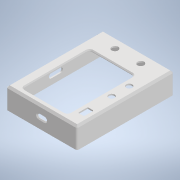
# Autodesk Inventor part: Frontpanel
Saved by Autodesk Inventor 2022 (Build 260153000, 153)
## iProperties
Created: 2020-11-05
Part Number: Frontpanel
Material: Generic
Document SubType Name: Modeling
Designer: simen
Density: 1 g/cm^3
Appearance: Default
Mass: 47.3769 g
Surface Area: 341.342 cm^2
Volume: 47.3769 cm^3
Author: simen
## iProperties of the stored document Frontpanel_3DPrint.ipt
Created: 2022-05-11
Part Number: Frontpanel_3DPrint
Material: Generic
Document SubType Name: Modeling
Designer: simen
Density: 1 g/cm^3
Appearance: Default
Author: simen
Autodesk Inventor part; units mm, degrees
ref_plane "YZ Plane" through (0, 0, 0) normal (1, 0, 0) x (0, 1, 0)
ref_plane "XZ Plane" through (0, 0, 0) normal (0, 1, 0) x (-1, 0, 0)
ref_plane "XY Plane" through (0, 0, 0) normal (0, 0, 1) x (1, 0, 0)
sketch "Sketch1" plane through (0, 0, 0) normal (0, 1, 0) x (-1, 0, 0)
  line L0 (-21.2777, 25.6513) -> (-98.2777, 25.6513)
  line L1 (-98.2777, 25.6513) -> (-98.2777, -79.3487)
  line L2 (-98.2777, -79.3487) -> (-21.2777, -79.3487)
  line L3 (-21.2777, -79.3487) -> (-21.2777, 25.6513)
  point P0 (0, 0)
  dimension "d0" = 77
  dimension "d42" = 105
  constraints: 8 end point, 2 parallel, 1 horizontal, 1 perpendicular
  measures "d0" distance of L2.end L1.end
  measures "d42" distance of L0.end L1.end
extrude "Extrusion1" add sketch "Sketch1" along normal blind 1.5
sketch "Sketch5" plane through (0, 0, 0) normal (0, -1, 0) x (1, 0, 0)
  line L0 (98.2777, 25.6513) -> (98.2777, -79.3487) projected
  line L1 (21.2777, 25.6513) -> (98.2777, 25.6513) projected
  line L2 (21.2777, -79.3487) -> (21.2777, 25.6513) projected
  line L3 (98.2777, -79.3487) -> (21.2777, -79.3487) projected
  line L4 (96.7777, 24.1513) -> (96.7777, -77.8487)
  line L5 (96.7777, -77.8487) -> (22.7777, -77.8487)
  line L6 (22.7777, -77.8487) -> (22.7777, 24.1513)
  line L7 (22.7777, 24.1513) -> (96.7777, 24.1513)
  point P0 (0, 0)
  dimension "d26" = 1.5
  constraints: 8 end point, 3 other
  measures "d26" distance between parallel lines of L1 L7
extrude "Extrusion7" add sketch "Sketch5" along normal blind 21.26
fillet "Fillet2" radius 2 4 edges at (21.2777, -9.88, -79.3487) (98.2777, -9.88, -79.3487) (98.2777, -9.88, 25.6513) (21.2777, -9.88, 25.6513)
sketch "Sketch8" plane through (21.2777, -21.26, -77.3487) normal (-1, 0, 0) x (0, 0, 1)
  line L0 (55.5, 8.76) -> (45.5, 8.76) construction
  line L1 (55.5, 11.26) -> (45.5, 11.26)
  line L2 (45.5, 6.26) -> (55.5, 6.26)
  arc A0 (55.5, 6.26) -> (55.5, 11.26) centre (55.5, 8.76) ccw
  arc A1 (45.5, 11.26) -> (45.5, 6.26) centre (45.5, 8.76) ccw
  line L3 (101, 0) -> (0, 0) projected
  line L4 (101, 0) -> (0, 0) construction
  line L5 (46.5661, 0) -> (44.4339, 17.52) construction
  line L6 (0, 22.76) -> (101, 22.76) projected
  line L7 (0, 22.76) -> (101, 22.76) construction
  line L8 (0, 0) -> (0, 22.76) construction
  line L9 (101, 22.76) -> (101, 0) projected
  line L10 (0, 0) -> (0, 22.76) projected
  circle A2 centre (50.054, 7.7768) radius 1.7526 projected
  point P0 (50.5, 8.76)
  point P1 (50.5, 8.76)
  dimension "d2" = 1.5
  dimension "d51" = 10
  dimension "d52" = 5
  dimension "d282" = 14
  constraints: 10 end point, 4 point on circle, 4 tangent, 2 centre point, 2 midpoint, 1 coincident, 1 horizontal, 1 parallel, 1 point on line
  measures "d51" distance of L0.end L0.start
  measures "d52" diameter of A1
  measures "d282" distance from line of L6 point (50.5, 8.76)
extrude "Extrusion9" cut sketch "Sketch8" against normal blind 10 contours A0 L2 A2 A1 L1 | L2 A2 picked at (50.5802, 7.7897)
sketch "Sketch9" plane through (0, 1.5, 0) normal (0, 1, 0) x (1, 0, 0)
  line L0 (35.2777, -19.1513) -> (78.2777, -19.1513)
  line L1 (81.2777, -16.1513) -> (81.2777, 50.8487)
  line L2 (78.2777, 53.8487) -> (35.2777, 53.8487)
  line L3 (32.2777, 50.8487) -> (32.2777, -16.1513)
  arc A0 (32.2777, -16.1513) -> (35.2777, -19.1513) centre (35.2777, -16.1513) ccw
  arc A1 (78.2777, -19.1513) -> (81.2777, -16.1513) centre (78.2777, -16.1513) ccw
  arc A2 (81.2777, 50.8487) -> (78.2777, 53.8487) centre (78.2777, 50.8487) ccw
  arc A3 (35.2777, 53.8487) -> (32.2777, 50.8487) centre (35.2777, 50.8487) ccw
  line L4 (98.2777, -25.6513) -> (98.2777, 79.3487) projected
  line L5 (21.2777, -25.6513) -> (98.2777, -25.6513) projected
  line L6 (22.7777, -24.1513) -> (22.7777, 77.8487) projected
  point P0 (0, 0)
  point P1 (81.2777, 53.8487)
  point P2 (81.2777, -19.1513)
  point P3 (32.2777, 53.8487)
  point P4 (98.2777, -23.6513)
  point P5 (98.2777, 77.3487)
  point P6 (23.2777, -25.6513)
  point P7 (96.2777, -25.6513)
  dimension "d56" = 49
  dimension "d57" = 73
  dimension "d60" = 3
  dimension "d116" = 17
  dimension "d144" = 6.5
  dimension "d283" = 9.5
  constraints: 8 end point, 8 point on circle, 8 tangent, 6 point on line, 4 centre point, 3 equal radius, 2 parallel, 1 horizontal, 1 perpendicular
  measures "d56" distance of point (32.278, 53.849) point (81.278, 53.849)
  measures "d57" distance of point (81.278, 53.849) point (81.278, -19.151)
  measures "d60" radius of A0
  measures "d116" distance between parallel lines of L4 L1
  measures "d144" distance between parallel lines of L5 L0
  measures "d283" distance between parallel lines of L6 L3
extrude "Extrusion10" cut sketch "Sketch9" against normal blind 10
chamfer "Chamfer4" distance 1 angle 45 8 edges at (33.1563, 1.5, 18.2726) (32.2777, 1.5, -17.3487) (33.1563, 1.5, -52.9701) (56.7777, 1.5, -53.8487) (80.399, 1.5, -52.9701) (81.2777, 1.5, -17.3487) (80.399, 1.5, 18.2726) (56.7777, 1.5, 19.1513)
chamfer "Chamfer5" distance 2 angle 45 8 edges at (98.2777, 1.5, -26.8487) (97.6919, 1.5, -78.763) (59.7777, 1.5, -79.3487) (21.8635, 1.5, -78.763) (21.2777, 1.5, -26.8487) (21.8635, 1.5, 25.0655) (59.7777, 1.5, 25.6513) (97.6919, 1.5, 25.0655)
sketch "Sketch17" plane through (23.2777, -21.26, 25.6513) normal (0, 0, 1) x (1, 0, 0)
  line L0 (0, 20.76) -> (73, 20.76) projected
  line L1 (73, 0) -> (0, 0) projected
  line L2 (33.5, 11.26) -> (39.5, 11.26) construction
  line L3 (33.5, 9.26) -> (39.5, 9.26)
  line L4 (39.5, 13.26) -> (33.5, 13.26)
  arc A0 (33.5, 13.26) -> (33.5, 9.26) centre (33.5, 11.26) ccw
  arc A1 (39.5, 9.26) -> (39.5, 13.26) centre (39.5, 11.26) ccw
  line L5 (0, 0) -> (0, 20.76) projected
  line L6 (73, 20.76) -> (73, 0) projected
  point P0 (-23.2777, 21.26)
  point P1 (36.5, 11.26)
  dimension "d167" = 6
  dimension "d168" = 4
  dimension "d169" = 9.5
  dimension "d170" = 11.26
  constraints: 8 end point, 4 point on circle, 4 tangent, 2 centre point, 1 horizontal, 1 midpoint, 1 parallel
  measures "d167" distance of L2.start L2.end
  measures "d168" diameter of A1
  measures "d169" distance between parallel lines of L0 L2
  measures "d170" distance from line of L1 point (36.5, 11.26)
extrude "Extrusion17" cut sketch "Sketch17" against normal blind 4 contours A0 L4 A1 L3
chamfer "Chamfer6" distance 1 angle 45 4 edges at (59.7777, -8, 25.6513) (64.7777, -10, 25.6513) (59.7777, -12, 25.6513) (54.7777, -10, 25.6513)
sketch "Sketch18" plane through (0, 1.5, 0) normal (0, 1, 0) x (1, 0, 0)
  line L0 (96.2777, 77.3487) -> (96.2777, -23.6513) projected
  line L1 (82.2777, -16.1513) -> (96.2777, -16.1513)
  line L2 (81.2777, 50.8487) -> (82.2777, 50.8487) projected
  line L3 (96.7777, -24.1513) -> (96.7777, 77.8487) projected
  circle A0 centre (88.7777, 21.3487) radius 3.25
  circle A1 centre (88.7777, 40.3987) radius 3.25
  line L4 (96.2777, -23.6513) -> (23.2777, -23.6513) projected
  point P0 (0, 0)
  point P1 (96.7777, -22.1513)
  point P2 (96.7777, 75.8487)
  point P3 (97.2777, 77.3487)
  point P4 (97.2777, -26.6513)
  dimension "d178" = 6.5
  dimension "d179" = 6.5
  dimension "d191" = 7.5
  dimension "d192" = 7.5
  dimension "d275" = 19.05
  dimension "d276" = 45
  constraints: 2 centre point, 2 end point, 1 horizontal, 2 other
  measures "d178" diameter of A0
  measures "d179" diameter of A1
  measures "d275" distance of A1.centre A0.centre
  measures "d276" distance from line of L4 A0.centre
extrude "Extrusion18" cut sketch "Sketch18" against normal blind 10
sketch "Sketch19" plane through (0, 1.5, 0) normal (0, 1, 0) x (1, 0, 0)
  circle A0 centre (88.7777, 40.3987) radius 3.25 projected
  circle A1 centre (88.7777, 21.3487) radius 3.25 projected
  arc A2 (31.2777, -16.1513) -> (35.2777, -20.1513) centre (35.2777, -16.1513) ccw projected
  line L0 (31.2777, 50.8487) -> (31.2777, -16.1513) projected
  arc A3 (35.2777, 54.8487) -> (31.2777, 50.8487) centre (35.2777, 50.8487) ccw projected
  line L1 (78.2777, 54.8487) -> (35.2777, 54.8487) projected
  arc A4 (82.2777, 50.8487) -> (78.2777, 54.8487) centre (78.2777, 50.8487) ccw projected
  line L2 (82.2777, -16.1513) -> (82.2777, 50.8487) projected
  arc A5 (78.2777, -20.1513) -> (82.2777, -16.1513) centre (78.2777, -16.1513) ccw projected
  line L3 (35.2777, -20.1513) -> (78.2777, -20.1513) projected
  line L4 (96.2777, -23.6513) -> (23.2777, -23.6513) projected
  line L5 (96.2777, 77.3487) -> (96.2777, -23.6513) projected
  line L6 (23.2777, 77.3487) -> (96.2777, 77.3487) projected
  line L7 (23.2777, -23.6513) -> (23.2777, 77.3487) projected
  arc A6 (35.2777, 54.8487) -> (31.2777, 50.8487) centre (35.2777, 50.8487) ccw projected
  arc A7 (82.2777, 50.8487) -> (78.2777, 54.8487) centre (78.2777, 50.8487) ccw projected
  line L8 (23.2777, 77.3487) -> (96.2777, 77.3487) projected
  circle A8 centre (73.7777, 67.8487) radius 3.5
  line L9 (96.2777, 77.3487) -> (96.2777, -23.6513) projected
  line L10 (81.2777, -16.1513) -> (81.2777, 50.8487) projected
  line L11 (88.7777, 40.3987) -> (88.7777, 73.4928)
  line L12 (96.7777, 75.8487) -> (96.7777, -22.1513) projected
  line L13 (24.7777, 77.8487) -> (94.7777, 77.8487) projected
  line L14 (82.2777, -16.1513) -> (82.2777, 50.8487) projected
  line L15 (82.2777, 43.5388) -> (96.2777, 43.5388)
  line L16 (87.0277, -12.4013) -> (91.5277, -12.4013)
  line L17 (92.5277, -11.4013) -> (92.5277, -2.9013)
  line L18 (91.5277, -1.9013) -> (87.0277, -1.9013)
  line L19 (86.0277, -2.9013) -> (86.0277, -11.4013)
  line L20 (86.0277, -12.4013) -> (92.5277, -1.9013) construction
  line L21 (92.5277, -12.4013) -> (86.0277, -1.9013) construction
  arc A9 (86.0277, -11.4013) -> (87.0277, -12.4013) centre (87.0277, -11.4013) ccw
  arc A10 (91.5277, -12.4013) -> (92.5277, -11.4013) centre (91.5277, -11.4013) ccw
  arc A11 (92.5277, -2.9013) -> (91.5277, -1.9013) centre (91.5277, -2.9013) ccw
  arc A12 (87.0277, -1.9013) -> (86.0277, -2.9013) centre (87.0277, -2.9013) ccw
  line L22 (77.1824, 62.3487) -> (70.6824, 72.8487) construction
  line L23 (35.0277, 59.5987) -> (41.5277, 70.0987) construction
  line L24 (98.2777, -23.6513) -> (98.2777, 77.3487) projected
  circle A13 centre (45.7777, 67.8487) radius 3.5
  line L25 (22.7777, -24.1513) -> (96.7777, -24.1513) projected
  point P0 (0, 0)
  point P1 (86.949, 59.6109)
  point P2 (88.2777, 58.5987)
  point P3 (89.2777, -7.1513)
  point P4 (98.2777, -25.6513)
  point P5 (98.2777, 79.3487)
  dimension "d184" = 7
  dimension "d200" = 10.5
  dimension "d201" = 1
  dimension "d207" = 6.5
  dimension "d209" = 5.75
  dimension "d277" = 7
  dimension "d278" = 28
  dimension "d284" = 9.5
  dimension "d285" = 9.5
  dimension "d286" = 22.5
  dimension "d318" = 17
  constraints: 20 end point, 11 point on line, 8 point on circle, 8 tangent, 6 centre point, 3 equal radius, 3 perpendicular, 2 parallel, 1 horizontal, 1 midpoint
  measures "d184" diameter of A8
  measures "d200" distance of L20.end L21.start
  measures "d201" radius of A9
  measures "d207" distance between parallel lines of L17 L19
  measures "d209" distance between parallel lines of L24 L17
  measures "d277" diameter of A13
  measures "d278" distance of A13.centre A8.centre
  measures "d284" distance from line of L6 A8.centre
  measures "d285" distance from line of L6 A13.centre
  measures "d286" distance from line of A13.centre L7
  measures "d318" distance from line of point (89.278, -7.151) L25
extrude "Extrusion19" cut sketch "Sketch19" against normal up to surface (1.5 mm away) contours A8 | A9 L19 A12 L18 A11 L17 A10 L16 | A13
sketch "Sketch34" plane through (0, 0, 0) normal (0, -1, 0) x (1, 0, 0)
  circle A0 centre (25.4777, 21.4513) radius 1.1
  circle A1 centre (25.4777, -75.1487) radius 1.1
  circle A2 centre (94.0777, -75.1487) radius 1.1
  circle A3 centre (94.0777, 21.4513) radius 1.1
  line L0 (22.7777, 24.1513) -> (96.7777, 24.1513) projected
  line L1 (96.7777, 24.1513) -> (96.7777, -77.8487) projected
  line L2 (22.7777, -14.9487) -> (22.7777, -38.7487)
  line L3 (96.7777, -77.8487) -> (22.7777, -77.8487) projected
  line L4 (22.7777, 24.1513) -> (22.7777, -77.8487) projected
  line L5 (24.7777, -75.8487) -> (94.7777, -75.8487)
  line L6 (94.7777, -75.8487) -> (94.7777, 22.1513)
  line L7 (94.7777, 22.1513) -> (24.7777, 22.1513)
  line L8 (24.7777, 22.1513) -> (24.7777, -75.8487)
  circle A4 centre (25.4777, -75.1487) radius 2.6
  circle A5 centre (25.4777, 21.4513) radius 2.6
  circle A6 centre (94.0777, -75.1487) radius 2.6
  circle A7 centre (94.0777, 21.4513) radius 2.6
  point P0 (0, 0)
  point P1 (27.4777, 19.4513)
  point P2 (92.0777, -73.1487)
  point P3 (24.7777, -72.6447)
  point P4 (24.7777, 18.9473)
  point P5 (27.9817, 22.1513)
  point P6 (91.5737, 22.1513)
  point P7 (94.7777, 18.9473)
  point P8 (94.7777, -72.6447)
  point P9 (91.5737, -75.8487)
  point P10 (27.9817, -75.8487)
  dimension "d361" = 2.2
  dimension "d362" = 2.2
  dimension "d363" = 2.2
  dimension "d364" = 2.2
  dimension "d367" = 2
  dimension "d368" = 1.5
  dimension "d369" = 1.5
  dimension "d370" = 1.5
  dimension "d371" = 1.5
  constraints: 10 end point, 8 centre point, 1 vertical, 5 other
  measures "d361" diameter of A0
  measures "d362" diameter of A1
  measures "d363" diameter of A2
  measures "d364" diameter of A3
  measures "d367" distance between parallel lines of L4 L8
  measures "d368" radial gap between concentric circles of A1 A4
  measures "d369" radial gap between concentric circles of A0 A5
  measures "d370" radial gap between concentric circles of A2 A6
  measures "d371" radial gap between concentric circles of A3 A7
fillet "Fillet6" radius 2 4 edges at (22.7777, -10.63, -77.8487) (22.7777, -10.63, 24.1513) (96.7777, -10.63, 24.1513) (96.7777, -10.63, -77.8487)
extrude "Extrusion31" add sketch "Sketch34" along normal blind 7 contours A0 L7 A5 L8 | A0 L8 A5 L7 | A7 L6 A3 L7 | L7 A3 L6 A7 | A4 L5 A1 L8 | L8 A1 L5 A4 | A6 L5 A2 L6 | L6 A2 L5 A6 | L0 L1 L3 L4 L2
sketch "Sketch35" plane through (0, -7, 0) normal (0, -1, 0) x (1, 0, 0)
  circle A0 centre (94.0777, 21.4513) radius 1.1 projected
  circle A1 centre (94.0777, -75.1487) radius 1.1 projected
  circle A2 centre (25.4777, 21.4513) radius 1.1 projected
  circle A3 centre (25.4777, -75.1487) radius 1.1 projected
  line L0 (24.7777, -72.6447) -> (24.7777, 18.9473) projected
  arc A4 (24.7777, 18.9473) -> (27.9817, 22.1513) centre (25.4777, 21.4513) ccw projected
  line L1 (27.9817, 22.1513) -> (91.5737, 22.1513) projected
  arc A5 (91.5737, 22.1513) -> (94.7777, 18.9473) centre (94.0777, 21.4513) ccw projected
  line L2 (94.7777, 18.9473) -> (94.7777, -72.6447) projected
  arc A6 (94.7777, -72.6447) -> (91.5737, -75.8487) centre (94.0777, -75.1487) ccw projected
  line L3 (91.5737, -75.8487) -> (27.9817, -75.8487) projected
  arc A7 (27.9817, -75.8487) -> (24.7777, -72.6447) centre (25.4777, -75.1487) ccw projected
  arc A8 (22.7777, -75.8487) -> (24.7777, -77.8487) centre (24.7777, -75.8487) ccw projected
  line L4 (94.7777, -77.8487) -> (24.7777, -77.8487) projected
  arc A9 (94.7777, -77.8487) -> (96.7777, -75.8487) centre (94.7777, -75.8487) ccw projected
  line L5 (96.7777, 22.1513) -> (96.7777, -75.8487) projected
  arc A10 (96.7777, 22.1513) -> (94.7777, 24.1513) centre (94.7777, 22.1513) ccw projected
  line L6 (24.7777, 24.1513) -> (94.7777, 24.1513) projected
  arc A11 (24.7777, 24.1513) -> (22.7777, 22.1513) centre (24.7777, 22.1513) ccw projected
  line L7 (22.7777, -75.8487) -> (22.7777, 22.1513) projected
  line L8 (24.7777, 24.1513) -> (94.7777, 24.1513) projected
  line L9 (34.7777, 24.1513) -> (34.7777, 22.1513)
  line L10 (27.9817, 22.1513) -> (91.5737, 22.1513) projected
  line L11 (28.7777, 22.1513) -> (28.7777, 24.1513)
  line L12 (84.2777, 24.1513) -> (84.2777, 22.1513)
  line L13 (78.2777, 24.1513) -> (78.2777, 22.1513)
  point P0 (0, 0)
  dimension "d372" = 6
  dimension "d373" = 6
  dimension "d374" = 6
  dimension "d375" = 10.5
  constraints: 8 end point, 8 point on line, 4 perpendicular
  measures "d372" distance between parallel lines of L9 L11
  measures "d373" distance between parallel lines of L7 L11
  measures "d374" distance between parallel lines of L12 L13
  measures "d375" distance between parallel lines of L2 L12
extrude "Extrusion32" cut sketch "Sketch35" against normal up to surface (7 mm away) contours L11 L6 L9 L1 | L13 L6 L12 L1
body "Solid1"
